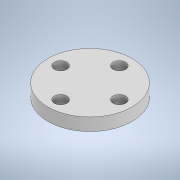
# Autodesk Inventor part: Twist_Servo_Horn
Saved by Autodesk Inventor 2022 (Build 260153000, 153)
## iProperties
Created: 2022-02-26
Part Number: Twist_Servo_Horn
Material: Generic
Document SubType Name: Modeling
Designer: Mlees
Density: 1 g/cm^3
Appearance: Default
Author: Mlees
Autodesk Inventor part; units mm, degrees
ref_plane "YZ Plane" through (0, 0, 0) normal (1, 0, 0) x (0, 1, 0)
ref_plane "XZ Plane" through (0, 0, 0) normal (0, 1, 0) x (-1, 0, 0)
ref_plane "XY Plane" through (0, 0, 0) normal (0, 0, 1) x (1, 0, 0)
sketch "Sketch1" plane through (0, 0, 0) normal (0, 1, 0) x (-1, 0, 0)
  circle A0 centre (0, 0) radius 10
  circle A1 centre (0, 0) radius 6.985
  circle A2 centre (6.985, 0) radius 1.5
  circle A3 centre (0, 6.985) radius 1.5
  circle A4 centre (-6.985, 0) radius 1.5
  circle A5 centre (0, -6.985) radius 1.5
  dimension "d1" = 13.97
  dimension "d0" = 20
  dimension "d2" = 3
  dimension "d5" = 360
  constraints: 5 centre point, 2 coincident, 1 horizontal alignment, 11 other
  measures "d0" diameter of A0
  measures "d2" diameter of A2
extrude "Extrusion1" add sketch "Sketch1" along normal blind 3 contours A0 | A2 A1 A5 A4 A3
body "Solid1"
